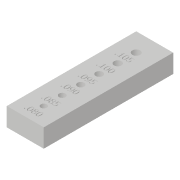
# Autodesk Inventor part: Screw thread test
Saved by Autodesk Inventor 2018 (Build 220112000, 112)
## iProperties
Created: 2019-09-26
Part Number: Screw thread test
Material: Generic
Document SubType Name: Modeling
Designer: ball
Density: 1 g/cm^3
Appearance: Default
Author: ball
Autodesk Inventor part; units mm, degrees
ref_plane "YZ Plane" through (0, 0, 0) normal (1, 0, 0) x (0, 1, 0)
ref_plane "XZ Plane" through (0, 0, 0) normal (0, 1, 0) x (-1, 0, 0)
ref_plane "XY Plane" through (0, 0, 0) normal (0, 0, 1) x (1, 0, 0)
sketch "Sketch1" plane through (0, 0, 0) normal (0, 1, 0) x (-1, 0, 0)
  line L0 (0, 0) -> (12.7, 0)
  line L1 (12.7, 0) -> (12.7, -44.45)
  line L2 (12.7, -44.45) -> (0, -44.45)
  line L3 (0, -44.45) -> (0, 0)
  circle A0 centre (6.35, -6.35) radius 1.016
  circle A1 centre (6.35, -12.7) radius 1.0795
  circle A2 centre (6.35, -19.05) radius 1.143
  circle A3 centre (6.35, -25.4) radius 1.2065
  circle A4 centre (6.35, -31.75) radius 1.27
  circle A5 centre (6.35, -38.1) radius 1.3335
  dimension "d0" = 12.7
  dimension "d2" = 2.032
  dimension "d3" = 6.35
  dimension "d4" = 6.35
  dimension "d5" = 2.159
  dimension "d6" = 2.286
  dimension "d7" = 2.413
  dimension "d8" = 2.54
  dimension "d9" = 2.667
  dimension "d10" = 6.35
  dimension "d11" = 6.35
  dimension "d12" = 6.35
  dimension "d13" = 6.35
  dimension "d14" = 6.35
  dimension "d15" = 6.35
  constraints: 8 end point, 6 centre point, 2 parallel, 1 horizontal, 1 perpendicular
  measures "d0" distance of L1.end L2.end
  measures "d2" diameter of A0
  measures "d3" distance from line of L3 A0.centre
  measures "d4" distance from line of L0 A0.centre
  measures "d5" diameter of A1
  measures "d6" diameter of A2
  measures "d7" diameter of A3
  measures "d8" diameter of A4
  measures "d9" diameter of A5
  measures "d10" distance of A0.centre A1.centre
  measures "d11" distance of A2.centre A1.centre
  measures "d12" distance of A2.centre A3.centre
  measures "d13" distance of A4.centre A3.centre
  measures "d14" distance of A5.centre A4.centre
  measures "d15" distance from line of L2 A5.centre
extrude "Extrusion1" add sketch "Sketch1" along normal blind 6.35
sketch "Sketch2" plane through (0, 6.35, 0) normal (0, 1, 0) x (1, 0, 0)
  line L0 (-9.3402, 4.2924) -> (-1.7583, 4.2924) construction
  line L1 (-1.7583, 4.2924) -> (-1.7583, 1.106) construction
  line L2 (-1.7583, 1.106) -> (-9.3402, 1.106) construction
  line L3 (-9.3402, 1.106) -> (-9.3402, 4.2924) construction
  line L4 (-9.4009, 10.2752) -> (-1.8191, 10.2752) construction
  line L5 (-1.8191, 10.2752) -> (-1.8191, 7.0889) construction
  line L6 (-1.8191, 7.0889) -> (-9.4009, 7.0889) construction
  line L7 (-9.4009, 7.0889) -> (-9.4009, 10.2752) construction
  line L8 (-9.599, 17.1509) -> (-2.0172, 17.1509) construction
  line L9 (-2.0172, 17.1509) -> (-2.0172, 13.9646) construction
  line L10 (-2.0172, 13.9646) -> (-9.599, 13.9646) construction
  line L11 (-9.599, 13.9646) -> (-9.599, 17.1509) construction
  line L12 (-9.6598, 23.0651) -> (-2.0779, 23.0651) construction
  line L13 (-2.0779, 23.0651) -> (-2.0779, 19.8788) construction
  line L14 (-2.0779, 19.8788) -> (-9.6598, 19.8788) construction
  line L15 (-9.6598, 19.8788) -> (-9.6598, 23.0651) construction
  line L16 (-9.7893, 29.5287) -> (-2.2074, 29.5287) construction
  line L17 (-2.2074, 29.5287) -> (-2.2074, 26.3424) construction
  line L18 (-2.2074, 26.3424) -> (-9.7893, 26.3424) construction
  line L19 (-9.7893, 26.3424) -> (-9.7893, 29.5287) construction
  line L20 (-9.85, 35.9237) -> (-2.2681, 35.9237) construction
  line L21 (-2.2681, 35.9237) -> (-2.2681, 32.7373) construction
  line L22 (-2.2681, 32.7373) -> (-9.85, 32.7373) construction
  line L23 (-9.85, 32.7373) -> (-9.85, 35.9237) construction
  line L24 (-8.7556, 2.2142) -> (-9.0816, 2.2142)
  line L25 (-9.0816, 2.2142) -> (-9.0816, 2.6029)
  line L26 (-9.0816, 2.6029) -> (-8.7556, 2.6029)
  line L27 (-8.7556, 2.6029) -> (-8.7556, 2.2142)
  spline S0 degree 2 poles (-7.0809, 3.2302) (-7.0809, 2.6836) (-7.3987, 2.1714) (-7.7297, 2.1714) knots 0 0 0 1 2 2 2
  spline S1 degree 2 poles (-7.7297, 2.1714) (-8.0656, 2.1714) (-8.3802, 2.6934) (-8.3802, 3.2286) knots 0 0 0 1 2 2 2
  spline S2 degree 2 poles (-8.3802, 3.2286) (-8.3802, 3.7786) (-8.0623, 4.2874) (-7.7297, 4.2874) knots 0 0 0 1 2 2 2
  spline S3 degree 2 poles (-7.7297, 4.2874) (-7.3954, 4.2874) (-7.0809, 3.7605) (-7.0809, 3.2302) knots 0 0 0 1 2 2 2
  spline S4 degree 2 poles (-7.43, 2.6111) (-7.3905, 2.7115) (-7.3576, 3.0211) (-7.3576, 3.2302) knots 0 0 0 1 2 2 2
  spline S5 degree 2 poles (-7.3576, 3.2302) (-7.3576, 3.4394) (-7.3905, 3.7473) (-7.4317, 3.851) knots 0 0 0 1 2 2 2
  spline S6 degree 2 poles (-7.4317, 3.851) (-7.4728, 3.9548) (-7.6161, 4.0618) (-7.7297, 4.0618) knots 0 0 0 1 2 2 2
  spline S7 degree 2 poles (-7.7297, 4.0618) (-7.8433, 4.0618) (-7.9899, 3.9548) (-8.0327, 3.8478) knots 0 0 0 1 2 2 2
  spline S8 degree 2 poles (-8.0327, 3.8478) (-8.0739, 3.744) (-8.1035, 3.4278) (-8.1035, 3.2286) knots 0 0 0 1 2 2 2
  spline S9 degree 2 poles (-8.1035, 3.2286) (-8.1035, 3.0145) (-8.0772, 2.728) (-8.0343, 2.616) knots 0 0 0 1 2 2 2
  spline S10 degree 2 poles (-8.0343, 2.616) (-7.9948, 2.5106) (-7.8483, 2.397) (-7.7297, 2.397) knots 0 0 0 1 2 2 2
  spline S11 degree 2 poles (-7.7297, 2.397) (-7.6177, 2.397) (-7.4712, 2.5041) (-7.43, 2.6111) knots 0 0 0 1 2 2 2
  spline S12 degree 2 poles (-6.2065, 2.1681) (-6.358, 2.1681) (-6.6067, 2.2587) (-6.694, 2.3427) knots 0 0 0 1 2 2 2
  spline S13 degree 2 poles (-6.694, 2.3427) (-6.7796, 2.425) (-6.8685, 2.649) (-6.8685, 2.7758) knots 0 0 0 1 2 2 2
  spline S14 degree 2 poles (-6.8685, 2.7758) (-6.8685, 2.9404) (-6.6923, 3.2171) (-6.5243, 3.2994) knots 0 0 0 1 2 2 2
  line L28 (-6.5243, 3.2994) -> (-6.5243, 3.3076)
  spline S15 degree 2 poles (-6.5243, 3.3076) (-6.6742, 3.3949) (-6.8191, 3.6024) (-6.8191, 3.7572) knots 0 0 0 1 2 2 2
  spline S16 degree 2 poles (-6.8191, 3.7572) (-6.8191, 3.9861) (-6.4733, 4.2924) (-6.2065, 4.2924) knots 0 0 0 1 2 2 2
  spline S17 degree 2 poles (-6.2065, 4.2924) (-5.9299, 4.2924) (-5.5956, 4.0025) (-5.5956, 3.7753) knots 0 0 0 1 2 2 2
  spline S18 degree 2 poles (-5.5956, 3.7753) (-5.5956, 3.6386) (-5.7553, 3.3719) (-5.9052, 3.2961) knots 0 0 0 1 2 2 2
  line L29 (-5.9052, 3.2961) -> (-5.9052, 3.2879)
  spline S19 degree 2 poles (-5.9052, 3.2879) (-5.7274, 3.2055) (-5.5446, 2.9684) (-5.5446, 2.7807) knots 0 0 0 1 2 2 2
  spline S20 degree 2 poles (-5.5446, 2.7807) (-5.5446, 2.5205) (-5.9233, 2.1681) (-6.2065, 2.1681) knots 0 0 0 1 2 2 2
  spline S21 degree 2 poles (-5.8245, 2.7544) (-5.8245, 2.8795) (-5.9233, 3.0277) (-6.0633, 3.1035) knots 0 0 0 1 2 2 2
  spline S22 degree 2 poles (-6.0633, 3.1035) (-6.1094, 3.1298) (-6.2642, 3.1907) (-6.3613, 3.2302) knots 0 0 0 1 2 2 2
  spline S23 degree 2 poles (-6.3613, 3.2302) (-6.4733, 3.1561) (-6.5935, 2.9355) (-6.5935, 2.7955) knots 0 0 0 1 2 2 2
  spline S24 degree 2 poles (-6.5935, 2.7955) (-6.5935, 2.6111) (-6.3712, 2.3707) (-6.2032, 2.3707) knots 0 0 0 1 2 2 2
  spline S25 degree 2 poles (-6.2032, 2.3707) (-6.032, 2.3707) (-5.8245, 2.5765) (-5.8245, 2.7544) knots 0 0 0 1 2 2 2
  spline S26 degree 2 poles (-5.8624, 3.772) (-5.8624, 3.9087) (-6.0452, 4.0915) (-6.2082, 4.0915) knots 0 0 0 1 2 2 2
  spline S27 degree 2 poles (-6.2082, 4.0915) (-6.3564, 4.0915) (-6.5458, 3.9284) (-6.5458, 3.7885) knots 0 0 0 1 2 2 2
  spline S28 degree 2 poles (-6.5458, 3.7885) (-6.5458, 3.688) (-6.4486, 3.5481) (-6.3514, 3.4921) knots 0 0 0 1 2 2 2
  spline S29 degree 2 poles (-6.3514, 3.4921) (-6.3103, 3.469) (-6.1357, 3.3883) (-6.0649, 3.3653) knots 0 0 0 1 2 2 2
  spline S30 degree 2 poles (-6.0649, 3.3653) (-5.9464, 3.4558) (-5.8624, 3.6485) (-5.8624, 3.772) knots 0 0 0 1 2 2 2
  spline S31 degree 2 poles (-4.0313, 3.2302) (-4.0313, 2.6836) (-4.3491, 2.1714) (-4.6801, 2.1714) knots 0 0 0 1 2 2 2
  spline S32 degree 2 poles (-4.6801, 2.1714) (-5.016, 2.1714) (-5.3305, 2.6934) (-5.3305, 3.2286) knots 0 0 0 1 2 2 2
  spline S33 degree 2 poles (-5.3305, 3.2286) (-5.3305, 3.7786) (-5.0127, 4.2874) (-4.6801, 4.2874) knots 0 0 0 1 2 2 2
  spline S34 degree 2 poles (-4.6801, 4.2874) (-4.3458, 4.2874) (-4.0313, 3.7605) (-4.0313, 3.2302) knots 0 0 0 1 2 2 2
  spline S35 degree 2 poles (-4.3804, 2.6111) (-4.3409, 2.7115) (-4.3079, 3.0211) (-4.3079, 3.2302) knots 0 0 0 1 2 2 2
  spline S36 degree 2 poles (-4.3079, 3.2302) (-4.3079, 3.4394) (-4.3409, 3.7473) (-4.382, 3.851) knots 0 0 0 1 2 2 2
  spline S37 degree 2 poles (-4.382, 3.851) (-4.4232, 3.9548) (-4.5664, 4.0618) (-4.6801, 4.0618) knots 0 0 0 1 2 2 2
  spline S38 degree 2 poles (-4.6801, 4.0618) (-4.7937, 4.0618) (-4.9402, 3.9548) (-4.9831, 3.8478) knots 0 0 0 1 2 2 2
  spline S39 degree 2 poles (-4.9831, 3.8478) (-5.0242, 3.744) (-5.0539, 3.4278) (-5.0539, 3.2286) knots 0 0 0 1 2 2 2
  spline S40 degree 2 poles (-5.0539, 3.2286) (-5.0539, 3.0145) (-5.0275, 2.728) (-4.9847, 2.616) knots 0 0 0 1 2 2 2
  spline S41 degree 2 poles (-4.9847, 2.616) (-4.9452, 2.5106) (-4.7986, 2.397) (-4.6801, 2.397) knots 0 0 0 1 2 2 2
  spline S42 degree 2 poles (-4.6801, 2.397) (-4.5681, 2.397) (-4.4215, 2.5041) (-4.3804, 2.6111) knots 0 0 0 1 2 2 2
  line L30 (-8.8164, 8.1971) -> (-9.1424, 8.1971)
  line L31 (-9.1424, 8.1971) -> (-9.1424, 8.5857)
  line L32 (-9.1424, 8.5857) -> (-8.8164, 8.5857)
  line L33 (-8.8164, 8.5857) -> (-8.8164, 8.1971)
  spline S43 degree 2 poles (-7.1417, 9.2131) (-7.1417, 8.6664) (-7.4595, 8.1543) (-7.7905, 8.1543) knots 0 0 0 1 2 2 2
  spline S44 degree 2 poles (-7.7905, 8.1543) (-8.1264, 8.1543) (-8.4409, 8.6763) (-8.4409, 9.2115) knots 0 0 0 1 2 2 2
  spline S45 degree 2 poles (-8.4409, 9.2115) (-8.4409, 9.7615) (-8.1231, 10.2703) (-7.7905, 10.2703) knots 0 0 0 1 2 2 2
  spline S46 degree 2 poles (-7.7905, 10.2703) (-7.4562, 10.2703) (-7.1417, 9.7433) (-7.1417, 9.2131) knots 0 0 0 1 2 2 2
  spline S47 degree 2 poles (-7.4908, 8.594) (-7.4513, 8.6944) (-7.4183, 9.004) (-7.4183, 9.2131) knots 0 0 0 1 2 2 2
  spline S48 degree 2 poles (-7.4183, 9.2131) (-7.4183, 9.4222) (-7.4513, 9.7302) (-7.4924, 9.8339) knots 0 0 0 1 2 2 2
  spline S49 degree 2 poles (-7.4924, 9.8339) (-7.5336, 9.9377) (-7.6769, 10.0447) (-7.7905, 10.0447) knots 0 0 0 1 2 2 2
  spline S50 degree 2 poles (-7.7905, 10.0447) (-7.9041, 10.0447) (-8.0507, 9.9377) (-8.0935, 9.8306) knots 0 0 0 1 2 2 2
  spline S51 degree 2 poles (-8.0935, 9.8306) (-8.1346, 9.7269) (-8.1643, 9.4107) (-8.1643, 9.2115) knots 0 0 0 1 2 2 2
  spline S52 degree 2 poles (-8.1643, 9.2115) (-8.1643, 8.9974) (-8.1379, 8.7109) (-8.0951, 8.5989) knots 0 0 0 1 2 2 2
  spline S53 degree 2 poles (-8.0951, 8.5989) (-8.0556, 8.4935) (-7.909, 8.3799) (-7.7905, 8.3799) knots 0 0 0 1 2 2 2
  spline S54 degree 2 poles (-7.7905, 8.3799) (-7.6785, 8.3799) (-7.5319, 8.4869) (-7.4908, 8.594) knots 0 0 0 1 2 2 2
  spline S55 degree 2 poles (-6.2673, 8.151) (-6.4188, 8.151) (-6.6674, 8.2416) (-6.7547, 8.3256) knots 0 0 0 1 2 2 2
  spline S56 degree 2 poles (-6.7547, 8.3256) (-6.8403, 8.4079) (-6.9293, 8.6318) (-6.9293, 8.7586) knots 0 0 0 1 2 2 2
  spline S57 degree 2 poles (-6.9293, 8.7586) (-6.9293, 8.9233) (-6.7531, 9.1999) (-6.5851, 9.2823) knots 0 0 0 1 2 2 2
  line L34 (-6.5851, 9.2823) -> (-6.5851, 9.2905)
  spline S58 degree 2 poles (-6.5851, 9.2905) (-6.735, 9.3778) (-6.8799, 9.5853) (-6.8799, 9.7401) knots 0 0 0 1 2 2 2
  spline S59 degree 2 poles (-6.8799, 9.7401) (-6.8799, 9.9689) (-6.5341, 10.2752) (-6.2673, 10.2752) knots 0 0 0 1 2 2 2
  spline S60 degree 2 poles (-6.2673, 10.2752) (-5.9907, 10.2752) (-5.6564, 9.9854) (-5.6564, 9.7582) knots 0 0 0 1 2 2 2
  spline S61 degree 2 poles (-5.6564, 9.7582) (-5.6564, 9.6215) (-5.8161, 9.3547) (-5.966, 9.279) knots 0 0 0 1 2 2 2
  line L35 (-5.966, 9.279) -> (-5.966, 9.2708)
  spline S62 degree 2 poles (-5.966, 9.2708) (-5.7881, 9.1884) (-5.6053, 8.9513) (-5.6053, 8.7636) knots 0 0 0 1 2 2 2
  spline S63 degree 2 poles (-5.6053, 8.7636) (-5.6053, 8.5034) (-5.9841, 8.151) (-6.2673, 8.151) knots 0 0 0 1 2 2 2
  spline S64 degree 2 poles (-5.8853, 8.7372) (-5.8853, 8.8624) (-5.9841, 9.0106) (-6.124, 9.0863) knots 0 0 0 1 2 2 2
  spline S65 degree 2 poles (-6.124, 9.0863) (-6.1701, 9.1127) (-6.3249, 9.1736) (-6.4221, 9.2131) knots 0 0 0 1 2 2 2
  spline S66 degree 2 poles (-6.4221, 9.2131) (-6.5341, 9.139) (-6.6543, 8.9184) (-6.6543, 8.7784) knots 0 0 0 1 2 2 2
  spline S67 degree 2 poles (-6.6543, 8.7784) (-6.6543, 8.594) (-6.432, 8.3536) (-6.264, 8.3536) knots 0 0 0 1 2 2 2
  spline S68 degree 2 poles (-6.264, 8.3536) (-6.0928, 8.3536) (-5.8853, 8.5594) (-5.8853, 8.7372) knots 0 0 0 1 2 2 2
  spline S69 degree 2 poles (-5.9231, 9.7549) (-5.9231, 9.8916) (-6.1059, 10.0743) (-6.2689, 10.0743) knots 0 0 0 1 2 2 2
  spline S70 degree 2 poles (-6.2689, 10.0743) (-6.4171, 10.0743) (-6.6065, 9.9113) (-6.6065, 9.7713) knots 0 0 0 1 2 2 2
  spline S71 degree 2 poles (-6.6065, 9.7713) (-6.6065, 9.6709) (-6.5094, 9.5309) (-6.4122, 9.4749) knots 0 0 0 1 2 2 2
  spline S72 degree 2 poles (-6.4122, 9.4749) (-6.371, 9.4519) (-6.1965, 9.3712) (-6.1257, 9.3481) knots 0 0 0 1 2 2 2
  spline S73 degree 2 poles (-6.1257, 9.3481) (-6.0071, 9.4387) (-5.9231, 9.6314) (-5.9231, 9.7549) knots 0 0 0 1 2 2 2
  spline S74 degree 2 poles (-4.125, 8.8426) (-4.125, 8.6961) (-4.2188, 8.4458) (-4.3045, 8.3536) knots 0 0 0 1 2 2 2
  spline S75 degree 2 poles (-4.3045, 8.3536) (-4.3901, 8.2613) (-4.6453, 8.1543) (-4.8034, 8.1543) knots 0 0 0 1 2 2 2
  spline S76 degree 2 poles (-4.8034, 8.1543) (-4.9483, 8.1543) (-5.2315, 8.2185) (-5.3353, 8.2696) knots 0 0 0 1 2 2 2
  line L36 (-5.3353, 8.2696) -> (-5.3353, 8.5577)
  line L37 (-5.3353, 8.5577) -> (-5.3155, 8.5577)
  spline S77 degree 2 poles (-5.3155, 8.5577) (-5.2842, 8.5347) (-5.1673, 8.4754) (-5.0965, 8.4491) knots 0 0 0 1 2 2 2
  spline S78 degree 2 poles (-5.0965, 8.4491) (-5.0158, 8.4211) (-4.8824, 8.3898) (-4.7985, 8.3898) knots 0 0 0 1 2 2 2
  spline S79 degree 2 poles (-4.7985, 8.3898) (-4.7161, 8.3898) (-4.5613, 8.4491) (-4.5054, 8.5133) knots 0 0 0 1 2 2 2
  spline S80 degree 2 poles (-4.5054, 8.5133) (-4.4543, 8.5742) (-4.4016, 8.7356) (-4.4016, 8.8443) knots 0 0 0 1 2 2 2
  spline S81 degree 2 poles (-4.4016, 8.8443) (-4.4016, 8.9529) (-4.4609, 9.0913) (-4.5169, 9.1374) knots 0 0 0 1 2 2 2
  spline S82 degree 2 poles (-4.5169, 9.1374) (-4.5745, 9.1884) (-4.7458, 9.2312) (-4.8495, 9.2312) knots 0 0 0 1 2 2 2
  spline S83 degree 2 poles (-4.8495, 9.2312) (-4.9615, 9.2312) (-5.1838, 9.1967) (-5.2513, 9.1818) knots 0 0 0 1 2 2 2
  line L38 (-5.2513, 9.1818) -> (-5.2513, 10.2291)
  line L39 (-5.2513, 10.2291) -> (-4.1365, 10.2291)
  line L40 (-4.1365, 10.2291) -> (-4.1365, 9.9904)
  line L41 (-4.1365, 9.9904) -> (-4.9895, 9.9904)
  line L42 (-4.9895, 9.9904) -> (-4.9895, 9.4486)
  spline S84 degree 2 poles (-4.9895, 9.4486) (-4.9401, 9.4552) (-4.8446, 9.4601) (-4.8051, 9.4601) knots 0 0 0 1 2 2 2
  spline S85 degree 2 poles (-4.8051, 9.4601) (-4.6486, 9.4601) (-4.4329, 9.4091) (-4.3341, 9.3333) knots 0 0 0 1 2 2 2
  spline S86 degree 2 poles (-4.3341, 9.3333) (-4.2337, 9.2576) (-4.125, 9.027) (-4.125, 8.8426) knots 0 0 0 1 2 2 2
  line L43 (-9.0145, 15.0777) -> (-9.3405, 15.0777)
  line L44 (-9.3405, 15.0777) -> (-9.3405, 15.4664)
  line L45 (-9.3405, 15.4664) -> (-9.0145, 15.4664)
  line L46 (-9.0145, 15.4664) -> (-9.0145, 15.0777)
  spline S87 degree 2 poles (-7.3398, 16.0937) (-7.3398, 15.547) (-7.6576, 15.0349) (-7.9886, 15.0349) knots 0 0 0 1 2 2 2
  spline S88 degree 2 poles (-7.9886, 15.0349) (-8.3245, 15.0349) (-8.639, 15.5569) (-8.639, 16.0921) knots 0 0 0 1 2 2 2
  spline S89 degree 2 poles (-8.639, 16.0921) (-8.639, 16.6421) (-8.3212, 17.1509) (-7.9886, 17.1509) knots 0 0 0 1 2 2 2
  spline S90 degree 2 poles (-7.9886, 17.1509) (-7.6543, 17.1509) (-7.3398, 16.624) (-7.3398, 16.0937) knots 0 0 0 1 2 2 2
  spline S91 degree 2 poles (-7.6889, 15.4746) (-7.6494, 15.575) (-7.6164, 15.8846) (-7.6164, 16.0937) knots 0 0 0 1 2 2 2
  spline S92 degree 2 poles (-7.6164, 16.0937) (-7.6164, 16.3029) (-7.6494, 16.6108) (-7.6905, 16.7145) knots 0 0 0 1 2 2 2
  spline S93 degree 2 poles (-7.6905, 16.7145) (-7.7317, 16.8183) (-7.875, 16.9253) (-7.9886, 16.9253) knots 0 0 0 1 2 2 2
  spline S94 degree 2 poles (-7.9886, 16.9253) (-8.1022, 16.9253) (-8.2488, 16.8183) (-8.2916, 16.7112) knots 0 0 0 1 2 2 2
  spline S95 degree 2 poles (-8.2916, 16.7112) (-8.3328, 16.6075) (-8.3624, 16.2913) (-8.3624, 16.0921) knots 0 0 0 1 2 2 2
  spline S96 degree 2 poles (-8.3624, 16.0921) (-8.3624, 15.878) (-8.336, 15.5915) (-8.2932, 15.4795) knots 0 0 0 1 2 2 2
  spline S97 degree 2 poles (-8.2932, 15.4795) (-8.2537, 15.3741) (-8.1072, 15.2605) (-7.9886, 15.2605) knots 0 0 0 1 2 2 2
  spline S98 degree 2 poles (-7.9886, 15.2605) (-7.8766, 15.2605) (-7.7301, 15.3676) (-7.6889, 15.4746) knots 0 0 0 1 2 2 2
  spline S99 degree 2 poles (-7.1356, 16.4494) (-7.1356, 16.6059) (-7.0335, 16.866) (-6.9446, 16.9599) knots 0 0 0 1 2 2 2
  spline S100 degree 2 poles (-6.9446, 16.9599) (-6.8606, 17.0505) (-6.6153, 17.1509) (-6.4901, 17.1509) knots 0 0 0 1 2 2 2
  spline S101 degree 2 poles (-6.4901, 17.1509) (-6.3502, 17.1509) (-6.1229, 17.057) (-6.0389, 16.9681) knots 0 0 0 1 2 2 2
  spline S102 degree 2 poles (-6.0389, 16.9681) (-5.9335, 16.8562) (-5.8183, 16.4939) (-5.8183, 16.2156) knots 0 0 0 1 2 2 2
  spline S103 degree 2 poles (-5.8183, 16.2156) (-5.8183, 15.9637) (-5.9319, 15.5125) (-6.0422, 15.3626) knots 0 0 0 1 2 2 2
  spline S104 degree 2 poles (-6.0422, 15.3626) (-6.1591, 15.2045) (-6.4885, 15.0382) (-6.7289, 15.0382) knots 0 0 0 1 2 2 2
  spline S105 degree 2 poles (-6.7289, 15.0382) (-6.7832, 15.0382) (-6.9067, 15.0497) (-6.9594, 15.0662) knots 0 0 0 1 2 2 2
  line L47 (-6.9594, 15.0662) -> (-6.9594, 15.328)
  line L48 (-6.9594, 15.328) -> (-6.9462, 15.328)
  spline S106 degree 2 poles (-6.9462, 15.328) (-6.9117, 15.3083) (-6.7668, 15.2737) (-6.6927, 15.2737) knots 0 0 0 1 2 2 2
  spline S107 degree 2 poles (-6.6927, 15.2737) (-6.4259, 15.2737) (-6.1213, 15.6261) (-6.0999, 15.9521) knots 0 0 0 1 2 2 2
  spline S108 degree 2 poles (-6.0999, 15.9521) (-6.2085, 15.878) (-6.4061, 15.8105) (-6.5231, 15.8105) knots 0 0 0 1 2 2 2
  spline S109 degree 2 poles (-6.5231, 15.8105) (-6.635, 15.8105) (-6.8211, 15.8599) (-6.915, 15.9307) knots 0 0 0 1 2 2 2
  spline S110 degree 2 poles (-6.915, 15.9307) (-7.0236, 16.0147) (-7.1356, 16.2699) (-7.1356, 16.4494) knots 0 0 0 1 2 2 2
  spline S111 degree 2 poles (-6.0933, 16.2765) (-6.0933, 16.4824) (-6.169, 16.7425) (-6.2365, 16.8133) knots 0 0 0 1 2 2 2
  spline S112 degree 2 poles (-6.2365, 16.8133) (-6.2958, 16.8792) (-6.4193, 16.9286) (-6.4918, 16.9286) knots 0 0 0 1 2 2 2
  spline S113 degree 2 poles (-6.4918, 16.9286) (-6.6597, 16.9286) (-6.859, 16.6882) (-6.859, 16.4609) knots 0 0 0 1 2 2 2
  spline S114 degree 2 poles (-6.859, 16.4609) (-6.859, 16.3325) (-6.7931, 16.1662) (-6.7207, 16.1069) knots 0 0 0 1 2 2 2
  spline S115 degree 2 poles (-6.7207, 16.1069) (-6.668, 16.0641) (-6.5379, 16.0361) (-6.4621, 16.0361) knots 0 0 0 1 2 2 2
  spline S116 degree 2 poles (-6.4621, 16.0361) (-6.3749, 16.0361) (-6.174, 16.097) (-6.0982, 16.1481) knots 0 0 0 1 2 2 2
  spline S117 degree 2 poles (-6.0982, 16.1481) (-6.0966, 16.1678) (-6.0933, 16.2354) (-6.0933, 16.2765) knots 0 0 0 1 2 2 2
  spline S118 degree 2 poles (-4.2902, 16.0937) (-4.2902, 15.547) (-4.608, 15.0349) (-4.939, 15.0349) knots 0 0 0 1 2 2 2
  spline S119 degree 2 poles (-4.939, 15.0349) (-5.2749, 15.0349) (-5.5894, 15.5569) (-5.5894, 16.0921) knots 0 0 0 1 2 2 2
  spline S120 degree 2 poles (-5.5894, 16.0921) (-5.5894, 16.6421) (-5.2716, 17.1509) (-4.939, 17.1509) knots 0 0 0 1 2 2 2
  spline S121 degree 2 poles (-4.939, 17.1509) (-4.6047, 17.1509) (-4.2902, 16.624) (-4.2902, 16.0937) knots 0 0 0 1 2 2 2
  spline S122 degree 2 poles (-4.6393, 15.4746) (-4.5997, 15.575) (-4.5668, 15.8846) (-4.5668, 16.0937) knots 0 0 0 1 2 2 2
  spline S123 degree 2 poles (-4.5668, 16.0937) (-4.5668, 16.3029) (-4.5997, 16.6108) (-4.6409, 16.7145) knots 0 0 0 1 2 2 2
  spline S124 degree 2 poles (-4.6409, 16.7145) (-4.6821, 16.8183) (-4.8253, 16.9253) (-4.939, 16.9253) knots 0 0 0 1 2 2 2
  spline S125 degree 2 poles (-4.939, 16.9253) (-5.0526, 16.9253) (-5.1991, 16.8183) (-5.2419, 16.7112) knots 0 0 0 1 2 2 2
  spline S126 degree 2 poles (-5.2419, 16.7112) (-5.2831, 16.6075) (-5.3127, 16.2913) (-5.3127, 16.0921) knots 0 0 0 1 2 2 2
  spline S127 degree 2 poles (-5.3127, 16.0921) (-5.3127, 15.878) (-5.2864, 15.5915) (-5.2436, 15.4795) knots 0 0 0 1 2 2 2
  spline S128 degree 2 poles (-5.2436, 15.4795) (-5.2041, 15.3741) (-5.0575, 15.2605) (-4.939, 15.2605) knots 0 0 0 1 2 2 2
  spline S129 degree 2 poles (-4.939, 15.2605) (-4.827, 15.2605) (-4.6804, 15.3676) (-4.6393, 15.4746) knots 0 0 0 1 2 2 2
  line L49 (-9.0752, 20.9919) -> (-9.4013, 20.9919)
  line L50 (-9.4013, 20.9919) -> (-9.4013, 21.3806)
  line L51 (-9.4013, 21.3806) -> (-9.0752, 21.3806)
  line L52 (-9.0752, 21.3806) -> (-9.0752, 20.9919)
  spline S130 degree 2 poles (-7.4006, 22.0079) (-7.4006, 21.4612) (-7.7184, 20.9491) (-8.0494, 20.9491) knots 0 0 0 1 2 2 2
  spline S131 degree 2 poles (-8.0494, 20.9491) (-8.3853, 20.9491) (-8.6998, 21.4711) (-8.6998, 22.0063) knots 0 0 0 1 2 2 2
  spline S132 degree 2 poles (-8.6998, 22.0063) (-8.6998, 22.5563) (-8.382, 23.0651) (-8.0494, 23.0651) knots 0 0 0 1 2 2 2
  spline S133 degree 2 poles (-8.0494, 23.0651) (-7.7151, 23.0651) (-7.4006, 22.5382) (-7.4006, 22.0079) knots 0 0 0 1 2 2 2
  spline S134 degree 2 poles (-7.7497, 21.3888) (-7.7101, 21.4892) (-7.6772, 21.7988) (-7.6772, 22.0079) knots 0 0 0 1 2 2 2
  spline S135 degree 2 poles (-7.6772, 22.0079) (-7.6772, 22.2171) (-7.7101, 22.525) (-7.7513, 22.6287) knots 0 0 0 1 2 2 2
  spline S136 degree 2 poles (-7.7513, 22.6287) (-7.7925, 22.7325) (-7.9357, 22.8395) (-8.0494, 22.8395) knots 0 0 0 1 2 2 2
  spline S137 degree 2 poles (-8.0494, 22.8395) (-8.163, 22.8395) (-8.3095, 22.7325) (-8.3523, 22.6254) knots 0 0 0 1 2 2 2
  spline S138 degree 2 poles (-8.3523, 22.6254) (-8.3935, 22.5217) (-8.4232, 22.2055) (-8.4232, 22.0063) knots 0 0 0 1 2 2 2
  spline S139 degree 2 poles (-8.4232, 22.0063) (-8.4232, 21.7922) (-8.3968, 21.5057) (-8.354, 21.3937) knots 0 0 0 1 2 2 2
  spline S140 degree 2 poles (-8.354, 21.3937) (-8.3145, 21.2883) (-8.1679, 21.1747) (-8.0494, 21.1747) knots 0 0 0 1 2 2 2
  spline S141 degree 2 poles (-8.0494, 21.1747) (-7.9374, 21.1747) (-7.7908, 21.2817) (-7.7497, 21.3888) knots 0 0 0 1 2 2 2
  spline S142 degree 2 poles (-7.1964, 22.3636) (-7.1964, 22.5201) (-7.0943, 22.7802) (-7.0054, 22.8741) knots 0 0 0 1 2 2 2
  spline S143 degree 2 poles (-7.0054, 22.8741) (-6.9214, 22.9647) (-6.676, 23.0651) (-6.5509, 23.0651) knots 0 0 0 1 2 2 2
  spline S144 degree 2 poles (-6.5509, 23.0651) (-6.4109, 23.0651) (-6.1837, 22.9712) (-6.0997, 22.8823) knots 0 0 0 1 2 2 2
  spline S145 degree 2 poles (-6.0997, 22.8823) (-5.9943, 22.7703) (-5.879, 22.4081) (-5.879, 22.1298) knots 0 0 0 1 2 2 2
  spline S146 degree 2 poles (-5.879, 22.1298) (-5.879, 21.8778) (-5.9927, 21.4267) (-6.103, 21.2768) knots 0 0 0 1 2 2 2
  spline S147 degree 2 poles (-6.103, 21.2768) (-6.2199, 21.1187) (-6.5492, 20.9524) (-6.7897, 20.9524) knots 0 0 0 1 2 2 2
  spline S148 degree 2 poles (-6.7897, 20.9524) (-6.844, 20.9524) (-6.9675, 20.9639) (-7.0202, 20.9804) knots 0 0 0 1 2 2 2
  line L53 (-7.0202, 20.9804) -> (-7.0202, 21.2422)
  line L54 (-7.0202, 21.2422) -> (-7.007, 21.2422)
  spline S149 degree 2 poles (-7.007, 21.2422) (-6.9724, 21.2225) (-6.8275, 21.1879) (-6.7534, 21.1879) knots 0 0 0 1 2 2 2
  spline S150 degree 2 poles (-6.7534, 21.1879) (-6.4867, 21.1879) (-6.182, 21.5403) (-6.1606, 21.8663) knots 0 0 0 1 2 2 2
  spline S151 degree 2 poles (-6.1606, 21.8663) (-6.2693, 21.7922) (-6.4669, 21.7247) (-6.5838, 21.7247) knots 0 0 0 1 2 2 2
  spline S152 degree 2 poles (-6.5838, 21.7247) (-6.6958, 21.7247) (-6.8819, 21.7741) (-6.9757, 21.8449) knots 0 0 0 1 2 2 2
  spline S153 degree 2 poles (-6.9757, 21.8449) (-7.0844, 21.9289) (-7.1964, 22.1841) (-7.1964, 22.3636) knots 0 0 0 1 2 2 2
  spline S154 degree 2 poles (-6.154, 22.1907) (-6.154, 22.3966) (-6.2298, 22.6567) (-6.2973, 22.7275) knots 0 0 0 1 2 2 2
  spline S155 degree 2 poles (-6.2973, 22.7275) (-6.3566, 22.7934) (-6.4801, 22.8428) (-6.5525, 22.8428) knots 0 0 0 1 2 2 2
  spline S156 degree 2 poles (-6.5525, 22.8428) (-6.7205, 22.8428) (-6.9197, 22.6024) (-6.9197, 22.3751) knots 0 0 0 1 2 2 2
  spline S157 degree 2 poles (-6.9197, 22.3751) (-6.9197, 22.2467) (-6.8539, 22.0804) (-6.7814, 22.0211) knots 0 0 0 1 2 2 2
  spline S158 degree 2 poles (-6.7814, 22.0211) (-6.7287, 21.9783) (-6.5986, 21.9503) (-6.5229, 21.9503) knots 0 0 0 1 2 2 2
  spline S159 degree 2 poles (-6.5229, 21.9503) (-6.4356, 21.9503) (-6.2347, 22.0112) (-6.159, 22.0623) knots 0 0 0 1 2 2 2
  spline S160 degree 2 poles (-6.159, 22.0623) (-6.1573, 22.082) (-6.154, 22.1495) (-6.154, 22.1907) knots 0 0 0 1 2 2 2
  spline S161 degree 2 poles (-4.3839, 21.6374) (-4.3839, 21.4909) (-4.4777, 21.2406) (-4.5633, 21.1484) knots 0 0 0 1 2 2 2
  spline S162 degree 2 poles (-4.5633, 21.1484) (-4.649, 21.0562) (-4.9042, 20.9491) (-5.0623, 20.9491) knots 0 0 0 1 2 2 2
  spline S163 degree 2 poles (-5.0623, 20.9491) (-5.2072, 20.9491) (-5.4904, 21.0133) (-5.5942, 21.0644) knots 0 0 0 1 2 2 2
  line L55 (-5.5942, 21.0644) -> (-5.5942, 21.3526)
  line L56 (-5.5942, 21.3526) -> (-5.5744, 21.3526)
  spline S164 degree 2 poles (-5.5744, 21.3526) (-5.5431, 21.3295) (-5.4262, 21.2702) (-5.3554, 21.2439) knots 0 0 0 1 2 2 2
  spline S165 degree 2 poles (-5.3554, 21.2439) (-5.2747, 21.2159) (-5.1413, 21.1846) (-5.0573, 21.1846) knots 0 0 0 1 2 2 2
  spline S166 degree 2 poles (-5.0573, 21.1846) (-4.975, 21.1846) (-4.8202, 21.2439) (-4.7642, 21.3081) knots 0 0 0 1 2 2 2
  spline S167 degree 2 poles (-4.7642, 21.3081) (-4.7132, 21.369) (-4.6605, 21.5304) (-4.6605, 21.6391) knots 0 0 0 1 2 2 2
  spline S168 degree 2 poles (-4.6605, 21.6391) (-4.6605, 21.7478) (-4.7198, 21.8861) (-4.7758, 21.9322) knots 0 0 0 1 2 2 2
  spline S169 degree 2 poles (-4.7758, 21.9322) (-4.8334, 21.9832) (-5.0047, 22.026) (-5.1084, 22.026) knots 0 0 0 1 2 2 2
  spline S170 degree 2 poles (-5.1084, 22.026) (-5.2204, 22.026) (-5.4427, 21.9915) (-5.5102, 21.9766) knots 0 0 0 1 2 2 2
  line L57 (-5.5102, 21.9766) -> (-5.5102, 23.0239)
  line L58 (-5.5102, 23.0239) -> (-4.3954, 23.0239)
  line L59 (-4.3954, 23.0239) -> (-4.3954, 22.7852)
  line L60 (-4.3954, 22.7852) -> (-5.2484, 22.7852)
  line L61 (-5.2484, 22.7852) -> (-5.2484, 22.2434)
  spline S171 degree 2 poles (-5.2484, 22.2434) (-5.199, 22.25) (-5.1035, 22.2549) (-5.0639, 22.2549) knots 0 0 0 1 2 2 2
  spline S172 degree 2 poles (-5.0639, 22.2549) (-4.9075, 22.2549) (-4.6918, 22.2039) (-4.593, 22.1281) knots 0 0 0 1 2 2 2
  spline S173 degree 2 poles (-4.593, 22.1281) (-4.4925, 22.0524) (-4.3839, 21.8219) (-4.3839, 21.6374) knots 0 0 0 1 2 2 2
  line L62 (-9.2047, 27.4555) -> (-9.5307, 27.4555)
  line L63 (-9.5307, 27.4555) -> (-9.5307, 27.8442)
  line L64 (-9.5307, 27.8442) -> (-9.2047, 27.8442)
  line L65 (-9.2047, 27.8442) -> (-9.2047, 27.4555)
  line L66 (-7.6436, 27.4555) -> (-8.6349, 27.4555)
  line L67 (-8.6349, 27.4555) -> (-8.6349, 27.663)
  line L68 (-8.6349, 27.663) -> (-8.2661, 27.663)
  line L69 (-8.2661, 27.663) -> (-8.2661, 29.0248)
  line L70 (-8.2661, 29.0248) -> (-8.6349, 29.0248)
  line L71 (-8.6349, 29.0248) -> (-8.6349, 29.2109)
  spline S174 degree 2 poles (-8.6349, 29.2109) (-8.4258, 29.2109) (-8.2282, 29.3295) (-8.215, 29.4941) knots 0 0 0 1 2 2 2
  line L72 (-8.215, 29.4941) -> (-8.0043, 29.4941)
  line L73 (-8.0043, 29.4941) -> (-8.0043, 27.663)
  line L74 (-8.0043, 27.663) -> (-7.6436, 27.663)
  line L75 (-7.6436, 27.663) -> (-7.6436, 27.4555)
  spline S175 degree 2 poles (-6.0052, 28.4715) (-6.0052, 27.9249) (-6.323, 27.4127) (-6.654, 27.4127) knots 0 0 0 1 2 2 2
  spline S176 degree 2 poles (-6.654, 27.4127) (-6.9899, 27.4127) (-7.3044, 27.9347) (-7.3044, 28.4699) knots 0 0 0 1 2 2 2
  spline S177 degree 2 poles (-7.3044, 28.4699) (-7.3044, 29.0199) (-6.9866, 29.5287) (-6.654, 29.5287) knots 0 0 0 1 2 2 2
  spline S178 degree 2 poles (-6.654, 29.5287) (-6.3197, 29.5287) (-6.0052, 29.0018) (-6.0052, 28.4715) knots 0 0 0 1 2 2 2
  spline S179 degree 2 poles (-6.3543, 27.8524) (-6.3148, 27.9528) (-6.2818, 28.2624) (-6.2818, 28.4715) knots 0 0 0 1 2 2 2
  spline S180 degree 2 poles (-6.2818, 28.4715) (-6.2818, 28.6807) (-6.3148, 28.9886) (-6.3559, 29.0923) knots 0 0 0 1 2 2 2
  spline S181 degree 2 poles (-6.3559, 29.0923) (-6.3971, 29.1961) (-6.5404, 29.3031) (-6.654, 29.3031) knots 0 0 0 1 2 2 2
  spline S182 degree 2 poles (-6.654, 29.3031) (-6.7676, 29.3031) (-6.9142, 29.1961) (-6.957, 29.0891) knots 0 0 0 1 2 2 2
  spline S183 degree 2 poles (-6.957, 29.0891) (-6.9981, 28.9853) (-7.0278, 28.6692) (-7.0278, 28.4699) knots 0 0 0 1 2 2 2
  spline S184 degree 2 poles (-7.0278, 28.4699) (-7.0278, 28.2558) (-7.0014, 27.9693) (-6.9586, 27.8573) knots 0 0 0 1 2 2 2
  spline S185 degree 2 poles (-6.9586, 27.8573) (-6.9191, 27.752) (-6.7725, 27.6383) (-6.654, 27.6383) knots 0 0 0 1 2 2 2
  spline S186 degree 2 poles (-6.654, 27.6383) (-6.542, 27.6383) (-6.3955, 27.7454) (-6.3543, 27.8524) knots 0 0 0 1 2 2 2
  spline S187 degree 2 poles (-4.4804, 28.4715) (-4.4804, 27.9249) (-4.7982, 27.4127) (-5.1292, 27.4127) knots 0 0 0 1 2 2 2
  spline S188 degree 2 poles (-5.1292, 27.4127) (-5.4651, 27.4127) (-5.7796, 27.9347) (-5.7796, 28.4699) knots 0 0 0 1 2 2 2
  spline S189 degree 2 poles (-5.7796, 28.4699) (-5.7796, 29.0199) (-5.4618, 29.5287) (-5.1292, 29.5287) knots 0 0 0 1 2 2 2
  spline S190 degree 2 poles (-5.1292, 29.5287) (-4.7949, 29.5287) (-4.4804, 29.0018) (-4.4804, 28.4715) knots 0 0 0 1 2 2 2
  spline S191 degree 2 poles (-4.8295, 27.8524) (-4.7899, 27.9528) (-4.757, 28.2624) (-4.757, 28.4715) knots 0 0 0 1 2 2 2
  spline S192 degree 2 poles (-4.757, 28.4715) (-4.757, 28.6807) (-4.7899, 28.9886) (-4.8311, 29.0923) knots 0 0 0 1 2 2 2
  spline S193 degree 2 poles (-4.8311, 29.0923) (-4.8723, 29.1961) (-5.0155, 29.3031) (-5.1292, 29.3031) knots 0 0 0 1 2 2 2
  spline S194 degree 2 poles (-5.1292, 29.3031) (-5.2428, 29.3031) (-5.3893, 29.1961) (-5.4321, 29.0891) knots 0 0 0 1 2 2 2
  spline S195 degree 2 poles (-5.4321, 29.0891) (-5.4733, 28.9853) (-5.503, 28.6692) (-5.503, 28.4699) knots 0 0 0 1 2 2 2
  spline S196 degree 2 poles (-5.503, 28.4699) (-5.503, 28.2558) (-5.4766, 27.9693) (-5.4338, 27.8573) knots 0 0 0 1 2 2 2
  spline S197 degree 2 poles (-5.4338, 27.8573) (-5.3943, 27.752) (-5.2477, 27.6383) (-5.1292, 27.6383) knots 0 0 0 1 2 2 2
  spline S198 degree 2 poles (-5.1292, 27.6383) (-5.0172, 27.6383) (-4.8706, 27.7454) (-4.8295, 27.8524) knots 0 0 0 1 2 2 2
  line L76 (-9.2654, 33.8505) -> (-9.5915, 33.8505)
  line L77 (-9.5915, 33.8505) -> (-9.5915, 34.2391)
  line L78 (-9.5915, 34.2391) -> (-9.2654, 34.2391)
  line L79 (-9.2654, 34.2391) -> (-9.2654, 33.8505)
  line L80 (-7.7044, 33.8505) -> (-8.6957, 33.8505)
  line L81 (-8.6957, 33.8505) -> (-8.6957, 34.058)
  line L82 (-8.6957, 34.058) -> (-8.3268, 34.058)
  line L83 (-8.3268, 34.058) -> (-8.3268, 35.4198)
  line L84 (-8.3268, 35.4198) -> (-8.6957, 35.4198)
  line L85 (-8.6957, 35.4198) -> (-8.6957, 35.6058)
  spline S199 degree 2 poles (-8.6957, 35.6058) (-8.4866, 35.6058) (-8.289, 35.7244) (-8.2758, 35.8891) knots 0 0 0 1 2 2 2
  line L86 (-8.2758, 35.8891) -> (-8.065, 35.8891)
  line L87 (-8.065, 35.8891) -> (-8.065, 34.058)
  line L88 (-8.065, 34.058) -> (-7.7044, 34.058)
  line L89 (-7.7044, 34.058) -> (-7.7044, 33.8505)
  spline S200 degree 2 poles (-6.066, 34.8665) (-6.066, 34.3198) (-6.3838, 33.8077) (-6.7147, 33.8077) knots 0 0 0 1 2 2 2
  spline S201 degree 2 poles (-6.7147, 33.8077) (-7.0507, 33.8077) (-7.3652, 34.3297) (-7.3652, 34.8648) knots 0 0 0 1 2 2 2
  spline S202 degree 2 poles (-7.3652, 34.8648) (-7.3652, 35.4148) (-7.0474, 35.9237) (-6.7147, 35.9237) knots 0 0 0 1 2 2 2
  spline S203 degree 2 poles (-6.7147, 35.9237) (-6.3805, 35.9237) (-6.066, 35.3967) (-6.066, 34.8665) knots 0 0 0 1 2 2 2
  spline S204 degree 2 poles (-6.415, 34.2473) (-6.3755, 34.3478) (-6.3426, 34.6574) (-6.3426, 34.8665) knots 0 0 0 1 2 2 2
  spline S205 degree 2 poles (-6.3426, 34.8665) (-6.3426, 35.0756) (-6.3755, 35.3835) (-6.4167, 35.4873) knots 0 0 0 1 2 2 2
  spline S206 degree 2 poles (-6.4167, 35.4873) (-6.4579, 35.591) (-6.6011, 35.6981) (-6.7147, 35.6981) knots 0 0 0 1 2 2 2
  spline S207 degree 2 poles (-6.7147, 35.6981) (-6.8284, 35.6981) (-6.9749, 35.591) (-7.0177, 35.484) knots 0 0 0 1 2 2 2
  spline S208 degree 2 poles (-7.0177, 35.484) (-7.0589, 35.3803) (-7.0885, 35.0641) (-7.0885, 34.8648) knots 0 0 0 1 2 2 2
  spline S209 degree 2 poles (-7.0885, 34.8648) (-7.0885, 34.6508) (-7.0622, 34.3643) (-7.0194, 34.2523) knots 0 0 0 1 2 2 2
  spline S210 degree 2 poles (-7.0194, 34.2523) (-6.9799, 34.1469) (-6.8333, 34.0333) (-6.7147, 34.0333) knots 0 0 0 1 2 2 2
  spline S211 degree 2 poles (-6.7147, 34.0333) (-6.6028, 34.0333) (-6.4562, 34.1403) (-6.415, 34.2473) knots 0 0 0 1 2 2 2
  spline S212 degree 2 poles (-4.5741, 34.496) (-4.5741, 34.3494) (-4.6679, 34.0991) (-4.7536, 34.0069) knots 0 0 0 1 2 2 2
  spline S213 degree 2 poles (-4.7536, 34.0069) (-4.8392, 33.9147) (-5.0944, 33.8077) (-5.2525, 33.8077) knots 0 0 0 1 2 2 2
  spline S214 degree 2 poles (-5.2525, 33.8077) (-5.3974, 33.8077) (-5.6806, 33.8719) (-5.7844, 33.9229) knots 0 0 0 1 2 2 2
  line L90 (-5.7844, 33.9229) -> (-5.7844, 34.2111)
  line L91 (-5.7844, 34.2111) -> (-5.7646, 34.2111)
  spline S215 degree 2 poles (-5.7646, 34.2111) (-5.7333, 34.1881) (-5.6164, 34.1288) (-5.5456, 34.1024) knots 0 0 0 1 2 2 2
  spline S216 degree 2 poles (-5.5456, 34.1024) (-5.4649, 34.0744) (-5.3315, 34.0431) (-5.2476, 34.0431) knots 0 0 0 1 2 2 2
  spline S217 degree 2 poles (-5.2476, 34.0431) (-5.1652, 34.0431) (-5.0104, 34.1024) (-4.9544, 34.1666) knots 0 0 0 1 2 2 2
  spline S218 degree 2 poles (-4.9544, 34.1666) (-4.9034, 34.2276) (-4.8507, 34.389) (-4.8507, 34.4976) knots 0 0 0 1 2 2 2
  spline S219 degree 2 poles (-4.8507, 34.4976) (-4.8507, 34.6063) (-4.91, 34.7446) (-4.966, 34.7907) knots 0 0 0 1 2 2 2
  spline S220 degree 2 poles (-4.966, 34.7907) (-5.0236, 34.8418) (-5.1949, 34.8846) (-5.2986, 34.8846) knots 0 0 0 1 2 2 2
  spline S221 degree 2 poles (-5.2986, 34.8846) (-5.4106, 34.8846) (-5.6329, 34.85) (-5.7004, 34.8352) knots 0 0 0 1 2 2 2
  line L92 (-5.7004, 34.8352) -> (-5.7004, 35.8825)
  line L93 (-5.7004, 35.8825) -> (-4.5856, 35.8825)
  line L94 (-4.5856, 35.8825) -> (-4.5856, 35.6437)
  line L95 (-4.5856, 35.6437) -> (-5.4386, 35.6437)
  line L96 (-5.4386, 35.6437) -> (-5.4386, 35.102)
  spline S222 degree 2 poles (-5.4386, 35.102) (-5.3892, 35.1085) (-5.2937, 35.1135) (-5.2541, 35.1135) knots 0 0 0 1 2 2 2
  spline S223 degree 2 poles (-5.2541, 35.1135) (-5.0977, 35.1135) (-4.882, 35.0624) (-4.7832, 34.9867) knots 0 0 0 1 2 2 2
  spline S224 degree 2 poles (-4.7832, 34.9867) (-4.6827, 34.9109) (-4.5741, 34.6804) (-4.5741, 34.496) knots 0 0 0 1 2 2 2
  point P0 (0, 0)
  constraints: 12 other
emboss "Emboss1" sketch "Sketch2" operation cut depth 0.762 direction (0, -1, 0)
body "Solid1"
